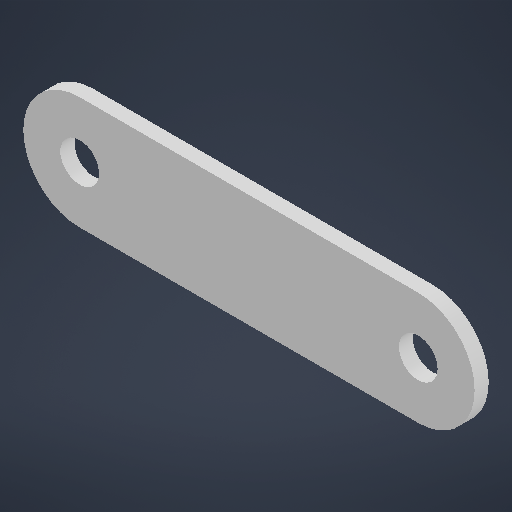
# Autodesk Inventor part: distancesensorcablemanage
Saved by Autodesk Inventor 2025.2 (Build 292293000, 293)
## iProperties
Created: 2025-01-26
Part Number: distancesensorcablemanage
Material: Generic
Document SubType Name: Modeling
Designer: Jahan
Density: 1 g/cm^3
Appearance: Default
Author: Jahan
Autodesk Inventor part; units mm, degrees
ref_plane "YZ Plane" through (0, 0, 0) normal (1, 0, 0) x (0, 1, 0)
ref_plane "XZ Plane" through (0, 0, 0) normal (0, 1, 0) x (-1, 0, 0)
ref_plane "XY Plane" through (0, 0, 0) normal (0, 0, 1) x (1, 0, 0)
sketch "Sketch1" plane through (0, 0, 0) normal (0, 0, 1) x (1, 0, 0)
  circle A0 centre (0, 0) radius 2.1844
  circle A1 centre (38.1, 0) radius 2.1844
  line L0 (0, 6.35) -> (38.1, 6.35)
  line L1 (38.1, -6.35) -> (0, -6.35)
  arc A2 (0, 6.35) -> (0, -6.35) centre (0, 0) ccw
  arc A3 (38.1, -6.35) -> (38.1, 6.35) centre (38.1, 0) ccw
  dimension "d0" = 4.3688
  dimension "d2" = 4.3688
  constraints: 4 centre point, 4 end point, 4 point on circle, 4 tangent, 1 coincident, 1 horizontal
  measures "d0" diameter of A0
  measures "d2" diameter of A1
extrude "Extrusion1" add sketch "Sketch1" along normal blind 1.5875
body "Solid1"
